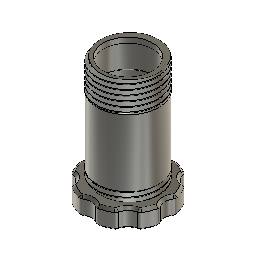
SPOOLadaptor (Autodesk Fusion 360 design; units mm, degrees)
Autodesk Fusion 360 part; units mm, degrees
sketch "Sketch1" plane through (0, 0, 0) normal (0, 0, 1) x (1, 0, 0)
  circle A0 centre (0, 0) radius 25
  circle A1 centre (0, 0) radius 20
  dimension "d1" = 50
  dimension "d34" = 40
  constraint coincident A0.centre A1.centre
  measures "d1" diameter of A0
  measures "d34" diameter of A1
extrude "Extrude1" add sketch "Sketch1" along normal blind 100 thin wall 5 inside contours A0 | A1 makes body 1
thread "Thread1" "ISO Metric profile 50.0 M50x4 6g" major diameter 49.7025 minor diameter 45.1258 pitch 4 angle 60 modelled right hand crest width 0.569 on face at (24.8758, -2.4892, 33.3333) crest through (24.8513, 0, -1) on bodies 1
extrude "Extrude2" add sketch "Sketch1" along normal blind 60 from surface at 20 thin wall 5 inside separate body contours A0 | A1 makes body 2
chamfer "Chamfer1" distance 3 angle 45 2 edges at (-23.3082, -9.0404, 20) (-23.3082, -9.0404, 80) on bodies 2
combine "Combine1" operation add target body 2 tool bodies 1
extrude "Extrude3" cut sketch "Sketch1" along normal blind 90 from surface at 5 thin wall 1 on the left open curves A1 bodies 2
extrude "Extrude4" cut sketch "Sketch1" along normal blind 50 from surface at 25 thin wall 3 outside contours A1 bodies 2
chamfer "Chamfer2" distance 1 angle 45 2 edges at (-18.6465, 7.2323, 95) (-18.6465, -7.2323, 5) on bodies 2
chamfer "Chamfer2" distance 2 angle 45 2 edges at (-19.5789, -7.5939, 25) (-19.5789, 7.5939, 75) on bodies 2
extrude "Extrude1'" add sketch "Sketch1" along normal blind 15 thin wall 8 outside separate body contours A0 | A1 makes body 3 in component "nut"
thread "Thread1'" "ISO Metric profile 50.0 M50x4 6H" major diameter 50.4462 minor diameter 45.9699 pitch 4 angle 60 modelled right hand crest width 1.0823 on face at (24.8758, -2.4892, 10) crest through (22.985, 0, 1) on bodies 3 in component "nut"
sketch "Sketch1 (2)" plane through (0, 0, 15) normal (0, 0, 1) x (-1, 0, 0) in component "nut"
  spline S0 degree 3 poles (15.169, -17.2687) (13.0004, -19.3661) (10.4399, -21.0156) (4.782, -23.2708) (1.7316, -23.8351) (-4.4707, -23.7724) (-7.5622, -23.1249) (-13.3792, -20.6688) (-16.0401, -18.8646) (-19.6742, -15.2049) (-20.8909, -13.6441) (-22.9418, -10.251) (-23.7645, -8.4283) (-24.3638, -6.5277) knots 0 0 0 0 0.905068 0.905068 1.826529 1.826529 2.764377 2.764377 3.718606 3.718606 4.309269 4.309269 4.906106 4.906106 4.906106 4.906106
  arc A0 (-24.3638, 6.5277) -> (-24.3638, -6.5277) centre (0, 0) ccw
  spline S1 degree 3 poles (-24.3638, 6.5277) (-23.3851, 9.6312) (-21.8146, 12.5156) (-17.6838, 17.471) (-15.1796, 19.5076) (-9.5754, 22.4714) (-6.5395, 23.3886) (-0.3409, 23.9919) (2.7598, 23.6933) (7.4915, 22.2689) (9.199, 21.5251) (12.3827, 19.6575) (13.8499, 18.5445) (15.169, 17.2687) knots 0 0 0 0 0.976263 0.976263 1.93612 1.93612 2.879566 2.879566 3.806595 3.806595 4.364231 4.364231 4.915681 4.915681 4.915681 4.915681
  arc A1 (15.169, -17.2687) -> (15.169, 17.2687) centre (0, 0) ccw
  circle A2 centre (0, -40) radius 10
  line L0 (0, -1.75) -> (0, -22.5)
  circle A3 centre (0, 0) radius 33
  dimension "d25" = 20
  dimension "d26" = 40
  constraint coincident A2.centre L0
  measures "d25" diameter of A2
  measures "d26" distance of A2.centre A0.centre
extrude "Extrude2'" cut sketch "Sketch1 (2)" against normal up to surface (15 mm away) contours A2 A3 | A2 A3 picked at (-0.2105, -38.6127) picked at (0, -31.9526) bodies 3 in component "nut"
fillet "Fillet3" radius 3 1 edges at (6.4551, 32.3625, 7.5) on bodies 3 in component "nut"
fillet "Fillet4" radius 3 1 edges at (-6.4551, 32.3625, 7.5) on bodies 3 in component "nut"
pattern_circular "C-Pattern1" count 8 over 360 about axis through (0, 0, 1.75) along (0, 0, 1) of "Extrude2'", "Fillet3", "Fillet4" in component "nut"
chamfer "Chamfer3" distance 2 angle 45 92 edges at (-21.2132, 21.2132, 0) (-18.004, 27.3837, 0) (-12.6286, 30.488, 0) (-6.6325, 32.0939, 0) (0, 30, 0) (6.6325, 32.0939, 0) (12.6286, 30.488, 0) (18.004, 27.3837, 0) (21.2132, 21.2132, 0) (27.3837, 18.004, 0) (30.488, 12.6286, 0) (32.0939, 6.6325, 0) (30, 0, 0) (32.0939, -6.6325, 0) (30.488, -12.6286, 0) (27.3837, -18.004, 0) (21.2132, -21.2132, 0) (18.004, -27.3837, 0) (12.6286, -30.488, 0) (6.6325, -32.0939, 0) (0, -30, 0) (-6.6325, -32.0939, 0) (-12.6286, -30.488, 0) (-18.004, -27.3837, 0) (-21.2132, -21.2132, 0) (-27.3837, -18.004, 0) (-30.488, -12.6286, 0) (-30.488, 12.6286, 0) (30.488, 12.6286, 0) (30.488, -12.6286, 0) (12.6286, -30.488, 0) (-12.6286, -30.488, 0) (-12.6286, 30.488, 0) (12.6286, 30.488, 0) (-32.0939, 6.6325, 0) (-30, 0, 0) (-32.0939, -6.6325, 0) (-30.488, -12.6286, 0) (-30.488, 12.6286, 0) (30.488, 12.6286, 0) (30.488, -12.6286, 0) (12.6286, -30.488, 0) (-12.6286, -30.488, 0) (-12.6286, 30.488, 0) (12.6286, 30.488, 0) (-27.3837, 18.004, 0) (-21.2132, 21.2132, 15) (-27.3837, 18.004, 15) (-30.488, 12.6286, 15) (-30.488, -12.6286, 15) (12.6286, 30.488, 15) (-12.6286, 30.488, 15) (-12.6286, -30.488, 15) (12.6286, -30.488, 15) (30.488, -12.6286, 15) (30.488, 12.6286, 15) (-32.0939, -6.6325, 15) (-30, 0, 15) (-32.0939, 6.6325, 15) (-30.488, 12.6286, 15) (-30.488, -12.6286, 15) (12.6286, 30.488, 15) (-12.6286, 30.488, 15) (-12.6286, -30.488, 15) (12.6286, -30.488, 15) (30.488, -12.6286, 15) (30.488, 12.6286, 15) (-27.3837, -18.004, 15) (-21.2132, -21.2132, 15) (-18.004, -27.3837, 15) (-12.6286, -30.488, 15) (-6.6325, -32.0939, 15) (0, -30, 15) (6.6325, -32.0939, 15) (12.6286, -30.488, 15) (18.004, -27.3837, 15) (21.2132, -21.2132, 15) (27.3837, -18.004, 15) (30.488, -12.6286, 15) (32.0939, -6.6325, 15) (30, 0, 15) (32.0939, 6.6325, 15) (30.488, 12.6286, 15) (27.3837, 18.004, 15) (21.2132, 21.2132, 15) (18.004, 27.3837, 15) (12.6286, 30.488, 15) (6.6325, 32.0939, 15) (0, 30, 15) (-6.6325, 32.0939, 15) (-12.6286, 30.488, 15) (-18.004, 27.3837, 15) on bodies 3 in component "nut"
component "nut" placed x (1, 0, 0) y (0, 1, 0) z (0, 0, 1) at (0, 0, 0)
named bodies: "shaftBody"
